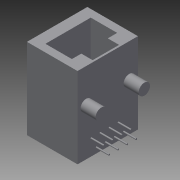
# Autodesk Inventor part: rj45
Saved by Autodesk Inventor 2015 (Build 190159000, 159)
## iProperties
Created: 2015-11-17
Part Number: rj45
Material: Generic
Document SubType Name: Modeling
Designer: Jufo
Density: 1 g/cm^3
Appearance: Default
Author: Jufo
Autodesk Inventor part; units mm, degrees
ref_plane "YZ Plane" through (0, 0, 0) normal (1, 0, 0) x (0, 1, 0)
ref_plane "XZ Plane" through (0, 0, 0) normal (0, 1, 0) x (-1, 0, 0)
ref_plane "XY Plane" through (0, 0, 0) normal (0, 0, 1) x (1, 0, 0)
sketch "Sketch1" plane through (0, 0, 0) normal (0, 1, 0) x (-1, 0, 0)
  line L0 (1.9169, 3.0365) -> (-11.4831, 3.0365)
  line L1 (-11.4831, 3.0365) -> (-11.4831, -12.9635)
  line L2 (-11.4831, -12.9635) -> (1.9169, -12.9635)
  line L3 (1.9169, -12.9635) -> (1.9169, 3.0365)
  point P0 (0, 0)
  dimension "d0" = 13.4
  dimension "d1" = 16
  constraints: 8 end point, 2 parallel, 1 horizontal, 1 perpendicular
  measures "d0" distance of L2.end L1.end
  measures "d1" distance of L1.end L0.end
extrude "Extrusion1" add sketch "Sketch1" along normal blind 21.4
sketch "Sketch2" plane through (0, 21.4, 0) normal (0, 1, 0) x (1, 0, 0)
  line L0 (0.9831, -1.0365) -> (0.9831, 10.9635)
  line L1 (11.4831, 12.9635) -> (-1.9169, 12.9635) projected
  line L2 (0.9831, 10.9635) -> (7.9831, 10.9635)
  line L3 (7.9831, 10.9635) -> (7.9831, 8.4635)
  line L4 (7.9831, 8.4635) -> (10.9831, 8.4635)
  line L5 (10.9831, 8.4635) -> (10.9831, 1.4635)
  line L6 (10.9831, 1.4635) -> (7.9831, 1.4635)
  line L7 (7.9831, 1.4635) -> (7.9831, -1.0365)
  line L8 (7.9831, -1.0365) -> (0.9831, -1.0365)
  line L9 (-1.9169, -3.0365) -> (11.4831, -3.0365) projected
  line L10 (-1.9169, 12.9635) -> (-1.9169, -3.0365) projected
  point P0 (0, 0)
  dimension "d4" = 12
  dimension "d5" = 7
  dimension "d6" = 7
  dimension "d7" = 3
  dimension "d8" = 7
  dimension "d9" = 2.5
  dimension "d10" = 2.5
  dimension "d11" = 2
  dimension "d12" = 2
  dimension "d13" = 2.9
  constraints: 16 end point, 7 perpendicular, 1 horizontal
  measures "d4" distance of L0.start L0.end
  measures "d5" distance of L0.end L2.end
  measures "d6" distance of L7.end L0.start
  measures "d7" distance of L5.end L6.end
  measures "d8" distance of L4.end L5.end
  measures "d9" distance of L2.end L3.end
  measures "d10" distance of L6.end L7.end
  measures "d11" distance between parallel lines of L1 L2
  measures "d12" distance between parallel lines of L9 L8
  measures "d13" distance between parallel lines of L0 L10
extrude "Extrusion2" cut sketch "Sketch2" against normal blind 12
sketch "Sketch3" plane through (11.4831, 0, 3.0365) normal (1, 0, 0) x (0, 0, -1)
  circle A0 centre (13.7, 12.4) radius 1.5
  circle A1 centre (2.3, 12.4) radius 1.5
  line L0 (0, 21.4) -> (16, 21.4) projected
  line L1 (0, 0) -> (0, 21.4) projected
  line L2 (16, 0) -> (16, 21.4) projected
  point P0 (3.0365, 0)
  dimension "d16" = 3
  dimension "d17" = 3
  dimension "d18" = 9
  dimension "d19" = 9
  dimension "d20" = 2.3
  dimension "d21" = 2.3
  constraints: 2 centre point
  measures "d16" diameter of A0
  measures "d17" diameter of A1
  measures "d18" distance from line of L0 A0.centre
  measures "d19" distance from line of L0 A1.centre
  measures "d20" distance from line of L1 A1.centre
  measures "d21" distance from line of L2 A0.centre
extrude "Extrusion3" add sketch "Sketch3" along normal blind 4
sketch "Sketch4" plane through (11.4831, 0, 3.0365) normal (1, 0, 0) x (0, 0, -1)
  circle A0 centre (3.6, 4.2) radius 0.2
  circle A1 centre (6, 4.2) radius 0.2
  line L0 (0, 0) -> (0, 21.4) projected
  circle A2 centre (8.4, 4.2) radius 0.2
  circle A3 centre (10.8, 4.2) radius 0.2
  line L1 (0, 0) -> (16, 0) projected
  line L2 (0.3816, 1.4) -> (15.1957, 1.4)
  circle A4 centre (5, 1.4) radius 0.2
  circle A5 centre (7.4, 1.4) radius 0.2
  circle A6 centre (9.8, 1.4) radius 0.2
  circle A7 centre (12.2, 1.4) radius 0.2
  point P0 (3.0365, 0)
  dimension "d24" = 0.4
  dimension "d25" = 0.4
  dimension "d26" = 3.6
  dimension "d27" = 2.4
  dimension "d28" = 0.4
  dimension "d29" = 0.4
  dimension "d30" = 2.4
  dimension "d31" = 2.4
  dimension "d32" = 0
  dimension "d33" = 0
  dimension "d34" = 0
  dimension "d35" = 4.2
  dimension "d36" = 1.4
  dimension "d37" = 0.4
  dimension "d38" = 0.4
  dimension "d39" = 0.4
  dimension "d40" = 0.4
  dimension "d41" = 1.4
  dimension "d42" = 2.4
  dimension "d43" = 2.4
  dimension "d44" = 2.4
  constraints: 8 centre point, 4 point on line, 2 end point, 1 horizontal
  measures "d24" diameter of A0
  measures "d25" diameter of A1
  measures "d26" distance from line of L0 A0.centre
  measures "d27" distance of A0.centre A1.centre
  measures "d28" diameter of A2
  measures "d29" diameter of A3
  measures "d30" distance of A1.centre A2.centre
  measures "d31" distance of A2.centre A3.centre
  measures "d32" vertical distance of A0.centre A1.centre
  measures "d33" vertical distance of A1.centre A2.centre
  measures "d34" vertical distance of A2.centre A3.centre
  measures "d35" distance from line of L1 A0.centre
  measures "d36" distance between parallel lines of L1 L2
  measures "d37" diameter of A4
  measures "d38" diameter of A5
  measures "d39" diameter of A6
  measures "d40" diameter of A7
  measures "d41" horizontal distance of A4.centre A0.centre
  measures "d42" distance between centres of A4 A5
  measures "d43" distance between centres of A5 A6
  measures "d44" distance between centres of A6 A7
extrude "Extrusion4" add sketch "Sketch4" along normal blind 3.4
equation "\"d21\" = d20"
body "Solid1"
